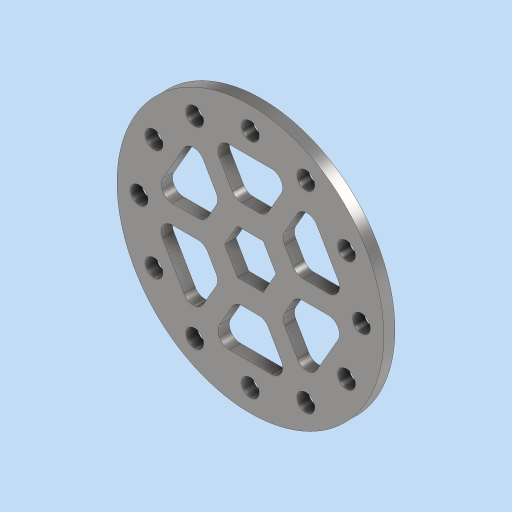
# Autodesk Inventor part: ThickWheelPlate_v8
Saved by Autodesk Inventor 2023 (Build 270158000, 158)
## iProperties
Created: 2023-04-06
Part Number: ThickWheelPlate_v8
Material: Steel, Alloy
Document SubType Name: Modeling
Designer: asach
Density: 7.73 g/cm^3
Appearance: Semi-Polished
Author: asach
Autodesk Inventor part; units mm, degrees
ref_plane "YZ Plane" through (0, 0, 0) normal (1, 0, 0) x (0, 1, 0)
ref_plane "XZ Plane" through (0, 0, 0) normal (0, 1, 0) x (-1, 0, 0)
ref_plane "XY Plane" through (0, 0, 0) normal (0, 0, 1) x (1, 0, 0)
sketch "Sketch1" plane through (0, 0, 0) normal (0, 0, 1) x (1, 0, 0)
  circle A0 centre (0, 0) radius 38.1
  line L0 (7.3323, 0) -> (3.6662, -6.35)
  line L1 (3.6662, -6.35) -> (-3.6662, -6.35)
  line L2 (-3.6662, -6.35) -> (-7.3323, 0)
  line L3 (-7.3323, 0) -> (-3.6662, 6.35)
  line L4 (-3.6662, 6.35) -> (3.6662, 6.35)
  line L5 (3.6662, 6.35) -> (7.3323, 0)
  circle A1 centre (0, 0) radius 31.75 construction
  circle A2 centre (0, 31.75) radius 2.4892
  circle A3 centre (-15.875, 27.4963) radius 2.4892
  circle A4 centre (-27.4963, 15.875) radius 2.4892
  circle A5 centre (-31.75, 0) radius 2.4892
  circle A6 centre (-27.4963, -15.875) radius 2.4892
  circle A7 centre (-15.875, -27.4963) radius 2.4892
  circle A8 centre (0, -31.75) radius 2.4892
  circle A9 centre (15.875, -27.4963) radius 2.4892
  circle A10 centre (27.4963, -15.875) radius 2.4892
  circle A11 centre (31.75, 0) radius 2.4892
  circle A12 centre (27.4963, 15.875) radius 2.4892
  circle A13 centre (15.875, 27.4963) radius 2.4892
  line L6 (-8.7971, 20.6375) -> (-5.1309, 14.2875)
  line L7 (-2.3812, 12.7) -> (2.3813, 12.7)
  line L8 (5.1309, 14.2875) -> (8.7971, 20.6375)
  line L9 (6.0474, 25.4) -> (-6.0474, 25.4)
  line L10 (0, -53.34) -> (0, 53.34) construction
  circle A14 centre (0, 0) radius 25.4 construction
  line L11 (0, 29.2608) -> (0, 25.4)
  line L12 (0, 38.1) -> (0, 25.4)
  arc A15 (-5.1309, 14.2875) -> (-2.3812, 12.7) centre (-2.3812, 15.875) ccw
  arc A16 (2.3813, 12.7) -> (5.1309, 14.2875) centre (2.3813, 15.875) ccw
  arc A17 (-6.0474, 25.4) -> (-8.7971, 20.6375) centre (-6.0474, 22.225) ccw
  arc A18 (8.7971, 20.6375) -> (6.0474, 25.4) centre (6.0474, 22.225) ccw
  point P0 (-11.5467, 25.4)
  point P1 (-4.2143, 12.7)
  point P2 (4.2143, 12.7)
  point P3 (11.5467, 25.4)
  dimension "d0" = 76.2
  dimension "d2" = 63.5
  dimension "d3" = 4.9784
  dimension "d1" = 12.7
  dimension "d6" = 360
  dimension "d16" = 6.35
  dimension "d20" = 12.7
  dimension "d21" = 60
  dimension "d23" = 3.175
  dimension "d24" = 3.175
  dimension "d25" = 4.7625
  constraints: 24 end point, 15 centre point, 10 point on line, 8 point on circle, 8 tangent, 4 coincident, 4 vertical alignment, 2 equal radius, 2 midpoint, 1 collinear, 1 equal length, 1 horizontal, 1 parallel, 1 perpendicular, 46 other
  measures "d1" distance between parallel lines of L1 L4
  measures "d16" distance between parallel lines of L4 L7
  measures "d20" distance of L12.start L11.end
  measures "d21" angle of L8 L6
  measures "d23" radius of A15
  measures "d24" radius of A17
  measures "d25" distance of A16.centre A15.centre
extrude "Extrusion1" add sketch "Sketch1" along normal blind 3.175 contours A0 | A17 L9 A18 L8 A16 L7 A15 L6
extrude "Extrusion2" cut sketch "Sketch1" along normal blind 3.175 contours A17 L9 A18 L8 A16 L7 A15 L6
fillet "Fillet1" [suppressed]
pattern_circular "Circular Pattern1" count 6 over 360 about axis through (0, 0, 0) along (0, 0, 1) of "Extrusion2"
body "Solid1"
